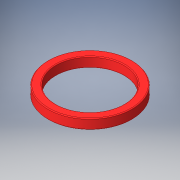
# Autodesk Inventor part: Button_ring_red
Saved by Autodesk Inventor 2016 (Build 200138000, 138)
## iProperties
Created: 2016-04-10
Part Number: Button_ring_red
Material: Acetal Resin, White
Document SubType Name: Modeling
Designer: agmle
Density: 1.425 g/cm^3
Appearance: Light Red
Author: agmle
Autodesk Inventor part; units mm, degrees
ref_plane "YZ Plane" through (0, 0, 0) normal (1, 0, 0) x (0, 1, 0)
ref_plane "XZ Plane" through (0, 0, 0) normal (0, 1, 0) x (-1, 0, 0)
ref_plane "XY Plane" through (0, 0, 0) normal (0, 0, 1) x (1, 0, 0)
sketch "Sketch1" plane through (0, 0, 0) normal (0, 1, 0) x (-1, 0, 0)
  circle A0 centre (0, 0) radius 5.25
  circle A1 centre (0, 0) radius 4.25
  dimension "d0" = 10.5
  dimension "d1" = 1
  constraints: 2 centre point, 2 coincident
  measures "d0" diameter of A0
  measures "d1" radial gap between concentric circles of A0 A1
extrude "Extrusion1" add sketch "Sketch1" along normal blind 1.25
fillet "Fillet1" radius 0.1 4 edges at (5.25, 1.25, 0) (4.25, 1.25, 0) (4.25, 0, 0) (5.25, 0, 0)
body "Solid1"
